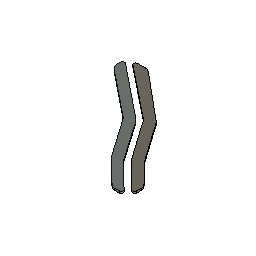
CNC_main (Autodesk Fusion 360 design; units mm, degrees)
Autodesk Fusion 360 part; units mm, degrees
note: some values were not read from the file. Chosen so that the rebuilt part matches the saved one: which bodies a step acts on.
sketch "Sketch1" plane through (0, 0, 0) normal (0, 0, 1) x (1, 0, 0)
  line L0 (0, 0) -> (300, 0)
  line L1 (0, 0) -> (0, 300)
  line L2 (0, 300) -> (300, 300)
  line L3 (300, 300) -> (300, 0)
  dimension "d1" = 300
  dimension "d2" = 300
  constraint coincident L0.start L1.start
  constraint horizontal L0
  constraint perpendicular L0 L1
  constraint perpendicular L1 L2
  constraint perpendicular L0 L3
  measures "d1" distance of L0.start L0.end
  measures "d2" distance of L0.start L1.end
extrude "Extrude1" add sketch "Sketch1" along normal blind 7 makes body 1
sketch "Sketch4" plane through (0, 0, 7) normal (0, 0, 1) x (-1, 0, 0)
sketch "Sketch5" plane through (0, 0, 7) normal (0, 0, 1) x (-1, 0, 0)
sketch "Sketch6" plane through (0, 0, 0) normal (0, 0, 1) x (1, 0, 0)
  line L0 (260, 0) -> (194.1266, 64.3484)
  line L1 (194.1266, 64.3484) -> (124.9116, 163.3043)
  line L2 (124.9116, 163.3043) -> (-0.0061, 263.7856)
  line L3 (-0.0061, 263.7856) -> (-0.0061, 291.7856)
  line L4 (-0.0061, 291.7856) -> (145.721, 174.5655)
  line L5 (145.721, 174.5655) -> (215.1743, 74.5568)
  line L6 (215.1743, 74.5568) -> (290, 0)
  line L7 (290, 0) -> (260, 0)
  dimension "d23" = 28
  constraint vertical L3
  constraint parallel L2 L4
  constraint horizontal L7
  measures "d23" distance of L2.end L3.end
sketch "Sketch7" plane through (0, 0, 0) normal (0, 0, 1) x (1, 0, 0)
  line L0 (300, 10) -> (225.0964, 83.7981)
  line L1 (225.0964, 83.7981) -> (154.1129, 184.833)
  line L2 (154.1129, 184.833) -> (10, 300)
  line L3 (10, 300) -> (50, 300)
  line L4 (50, 300) -> (175.3562, 195.7137)
  line L5 (175.3562, 195.7137) -> (245.6085, 95.7195)
  line L6 (245.6085, 95.7195) -> (300, 40)
  line L7 (300, 40) -> (300, 10)
  constraint horizontal L3
  constraint parallel L1 L5
  constraint vertical L7
extrude "Extrude2" add sketch "Sketch7" against normal blind 5 bodies 1
extrude "Extrude3" add sketch "Sketch6" against normal blind 5 bodies 1
extrude "Extrude4" cut 1 faces at (100, 200, 7) along direction (0, 0, -1) blind 7 on bodies 1 bodies 1 makes body 2 at (154.9197, 134.0727, -5)
fillet "Fillet1" radius 15 1 edges at (260, 0, -2.5) on bodies 2
fillet "Fillet2" radius 15 1 edges at (194.1266, 64.3484, -2.5) on bodies 2
fillet "Fillet3" radius 15 1 edges at (124.9116, 163.3043, -2.5) on bodies 2
fillet "Fillet4" radius 15 1 edges at (-0.0061, 263.7856, -2.5) on bodies 2
fillet "Fillet5" radius 15 1 edges at (50, 300, -2.5) on bodies 1
fillet "Fillet6" radius 15 1 edges at (175.3562, 195.7137, -2.5) on bodies 1
fillet "Fillet7" radius 15 1 edges at (245.6085, 95.7195, -2.5) on bodies 1
fillet "Fillet8" radius 15 1 edges at (300, 40, -2.5) on bodies 1
fillet "Fillet9" radius 15 1 edges at (215.1743, 74.5568, -2.5) on bodies 2
fillet "Fillet10" radius 15 1 edges at (145.721, 174.5655, -2.5) on bodies 2
fillet "Fillet11" radius 15 1 edges at (154.1129, 184.833, -2.5) on bodies 1
fillet "Fillet12" radius 15 1 edges at (225.0964, 83.7981, -2.5) on bodies 1
sketch "Sketch8" plane through (0, 0, 0) normal (0, 0, 1) x (1, 0, 0)
fillet "Fillet13" radius 5 1 edges at (290, 0, -2.5) on bodies 2
fillet "Fillet14" radius 5 1 edges at (300, 10, -2.5) on bodies 1
fillet "Fillet15" radius 5 1 edges at (-0.0061, 291.7856, -2.5) on bodies 2
fillet "Fillet16" radius 5 1 edges at (10, 300, -2.5) on bodies 1
sketch "Sketch9" plane through (0, 0, 0) normal (0, 0, 1) x (-1, 0, 0)
  arc A0 (-8.1278, -285.2429) -> (0.0061, -281.3469) centre (-4.9939, -281.3469) ccw
  line L0 (0.0061, -281.3469) -> (0.0061, -270.9704)
  arc A1 (0.0061, -270.9704) -> (-5.5923, -259.2824) centre (-14.9939, -270.9704) ccw
  line L1 (-5.5923, -259.2824) -> (-123.2464, -164.6437)
  arc A2 (-126.1364, -161.5531) -> (-123.2464, -164.6437) centre (-113.8448, -152.9557) ccw
  line L2 (-126.1364, -161.5531) -> (-193.3215, -65.4995)
  arc A3 (-193.3215, -65.4995) -> (-195.1315, -63.3668) centre (-205.6131, -74.0969) ccw
  line L3 (-195.1315, -63.3668) -> (-255.6289, -4.2699)
  arc A4 (-255.6289, -4.2699) -> (-266.1106, 0) centre (-266.1106, -15) ccw
  line L4 (-266.1106, 0) -> (-277.8981, 0)
  arc A5 (-277.8981, 0) -> (-281.4273, -8.5419) centre (-277.8981, -5) ccw
  line L5 (-281.4273, -8.5419) -> (-216.1343, -73.6003)
  arc A6 (-214.4014, -75.6698) -> (-216.1343, -73.6003) centre (-226.7218, -84.226) ccw
  line L6 (-214.4014, -75.6698) -> (-146.9546, -172.7892)
  arc A7 (-146.9546, -172.7892) -> (-144.0359, -175.921) centre (-134.6343, -164.233) ccw
  line L7 (-144.0359, -175.921) -> (-8.1278, -285.2429)
